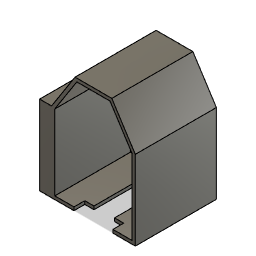
dc-15s_custom_holster (Autodesk Fusion 360 design; units mm, degrees)
Autodesk Fusion 360 part; units mm, degrees
sketch "Sketch1" plane through (0, 0, 0) normal (0, 1, 0) x (1, 0, 0)
other "Base Mesh Feature1"
other "Base Mesh Feature2"
sketch "Sketch2" plane through (0, 0, 0) normal (0, 0, 1) x (1, 0, 0)
  line L0 (-38.75, -35) -> (38.75, -35)
  line L1 (38.75, -35) -> (38.75, 35)
  line L2 (38.75, 35) -> (-38.75, 35)
  line L3 (-38.75, 35) -> (-38.75, -35)
  line L4 (-38.75, -35) -> (38.75, 35) construction
  line L5 (38.75, -35) -> (-38.75, 35) construction
  line L6 (38.75, 35) -> (-38.75, 35)
  line L7 (-38.75, 35) -> (-38.75, 47.5)
  line L8 (-38.75, 47.5) -> (38.75, 47.5)
  line L9 (38.75, 47.5) -> (38.75, 35)
  line L10 (25, 58.75) -> (-25, 58.75)
  line L11 (-25, 58.75) -> (-25, 11.25)
  line L12 (-25, 11.25) -> (25, 11.25)
  line L13 (25, 11.25) -> (25, 58.75)
  line L14 (25, 58.75) -> (-25, 11.25) construction
  line L15 (-25, 58.75) -> (25, 11.25) construction
  line L16 (17, 0.41) -> (-17, 0.41)
  line L17 (-17, 0.41) -> (-17, 69.59)
  line L18 (-17, 69.59) -> (17, 69.59)
  line L19 (17, 69.59) -> (17, 0.41)
  line L20 (17, 0.41) -> (-17, 69.59) construction
  line L21 (-17, 0.41) -> (17, 69.59) construction
  line L22 (25, 35) -> (17, 47.5)
  line L23 (-17, 47.5) -> (-25, 35)
  line L24 (38.75, -35) -> (-38.75, -35)
  line L25 (-38.75, -35) -> (-38.75, -60)
  line L26 (-38.75, -60) -> (38.75, -60)
  line L27 (38.75, -60) -> (38.75, -35)
  line L28 (-17, 47.5) -> (-38.75, 13.5156)
  line L29 (17, 47.5) -> (38.75, 13.5156)
  point P0 (0, 35)
  point P1 (0, 35)
  dimension "d1" = 77.5
  dimension "d2" = 70
  dimension "d3" = 12.5
  dimension "d4" = 50
  dimension "d5" = 47.5
  dimension "d6" = 34
  dimension "d7" = 25
  constraint horizontal L0
  constraint perpendicular L0 L1
  constraint parallel L0 L2
  constraint parallel L1 L3
  constraint coincident L4 origin
  constraint coincident L5 origin
  constraint perpendicular L6 L7
  constraint parallel L6 L8
  constraint parallel L7 L9
  constraint horizontal L10
  constraint perpendicular L10 L11
  constraint parallel L10 L12
  constraint parallel L11 L13
  constraint coincident L14 P1
  constraint coincident L15 P1
  constraint midpoint L6 P1
  constraint horizontal L16
  constraint perpendicular L16 L17
  constraint parallel L16 L18
  constraint parallel L17 L19
  constraint coincident L20 P1
  constraint coincident L21 P1
  constraint coincident P1 P0
  constraint midpoint L13 L22.start
  constraint coincident L8 L22.end
  constraint coincident L19 L22.end
  constraint coincident L8 L23.start
  constraint coincident L17 L23.start
  constraint midpoint L11 L23.end
  constraint perpendicular L24 L25
  constraint parallel L24 L26
  constraint parallel L25 L27
  constraint parallel L23 L28
  constraint coincident L1 L29.end
  constraint parallel L22 L29
  measures "d1" distance of L1.end L2.end
  measures "d2" distance of L0.end L1.end
  measures "d3" distance of L1.end L8.end
  measures "d4" distance of L11.end L12.end
  measures "d5" distance of L10.end L11.end
  measures "d6" distance of L17.end L18.end
  measures "d7" distance of L0.end L26.end
extrude "Extrude1" add sketch "Sketch2" along normal blind 5 contours L0 L1 L3 L11 L12 L13 L16 L17 L19 L24 L28 L29 | L0 L24 L25 L26 L27 | L2 L6 L17 L23 L28 | L2 L6 L11 L12 L17 | L2 L6 L12 L13 L19 | L2 L6 L19 L22 L29 | L2 L6 L8 L17 L19 | L2 L6 L12 L17 L19 | L12 L16 L17 L19
sketch "Sketch3" plane through (0, 0, 5) normal (0, 0, 1) x (1, 0, 0)
  line L0 (38.75, 13.5156) -> (17, 47.5)
  line L1 (17, 47.5) -> (-17, 47.5)
  line L2 (-17, 47.5) -> (-38.75, 13.5156)
  line L3 (-38.75, 13.5156) -> (-38.75, -60)
  line L4 (38.75, -60) -> (38.75, 13.5156)
  line L5 (-38.75, -60) -> (38.75, -60)
  line L6 (23.3582, 32) -> (15.3582, 44.5)
  line L7 (15.3582, 44.5) -> (-15.3582, 44.5)
  line L8 (-15.3582, 44.5) -> (-23.3582, 32)
  line L9 (-23.3582, 32) -> (-35.75, 32)
  line L10 (-35.75, 32) -> (-35.75, -57)
  line L11 (-35.75, -57) -> (35.75, -57)
  line L12 (35.75, -57) -> (35.75, 32)
  line L13 (35.75, 32) -> (23.3582, 32)
  line L14 (-15.3582, 44.5) -> (-35.75, 12.6378)
  line L15 (15.3582, 44.5) -> (35.75, 12.6378)
  constraint parallel L0 L6
  constraint parallel L1 L7
  constraint parallel L2 L8
  constraint parallel L3 L10
  constraint parallel L5 L11
  constraint parallel L4 L12
  constraint coincident L10 L14.end
  constraint parallel L2 L14
  constraint coincident L12 L15.end
  constraint parallel L6 L15
extrude "Extrude2" add sketch "Sketch3" along normal blind 10 contours L0 L2 L3 L4 L5 L10 L11 L12 | L0 L12 L13 L15 | L0 L1 L2 L6 L7 L8 L9 L13 L14 L15 | L2 L9 L10 L14
sketch "Sketch4" plane through (0, 0, 15) normal (0, 0, 1) x (1, 0, 0)
  line L0 (35.75, 12.6378) -> (35.75, -57)
  line L1 (35.75, -57) -> (-35.75, -57)
  line L2 (-35.75, -57) -> (-35.75, 12.6378)
  line L3 (-38.75, -60) -> (38.75, -60)
  line L4 (38.75, -60) -> (38.75, 13.5156)
  line L5 (38.75, 13.5156) -> (17, 47.5)
  line L6 (-17, 47.5) -> (-38.75, 13.5156)
  line L7 (-38.75, 13.5156) -> (-38.75, -60)
  line L8 (9.5, -63.0415) -> (-9.5, -63.0415)
  line L9 (-9.5, -63.0415) -> (-9.5, -56.9585)
  line L10 (-9.5, -56.9585) -> (9.5, -56.9585)
  line L11 (9.5, -56.9585) -> (9.5, -63.0415)
  line L12 (9.5, -63.0415) -> (-9.5, -56.9585) construction
  line L13 (-9.5, -63.0415) -> (9.5, -56.9585) construction
  line L14 (-35.75, 12.6378) -> (-15.3582, 44.5)
  line L15 (-15.3582, 44.5) -> (15.3582, 44.5)
  line L16 (15.3582, 44.5) -> (35.75, 12.6378)
  line L17 (17, 47.5) -> (-17, 47.5)
  point P0 (0, -60)
  dimension "d14" = 19
  constraint horizontal L8
  constraint perpendicular L8 L9
  constraint parallel L8 L10
  constraint parallel L9 L11
  constraint coincident L12 P0
  constraint coincident L13 P0
  constraint midpoint L3 P0
  measures "d14" distance of L9.end L10.end
extrude "Extrude3" add sketch "Sketch4" along normal blind 50 contours L0 L1 L2 L3 L4 L5 L6 L7 L9 L11 L14 L15 L16 L17
sketch "Sketch5" plane through (0, 0, 5) normal (0, 0, 1) x (1, 0, 0)
  line L0 (-35.75, 12.6378) -> (-35.75, -57)
  line L1 (-35.75, -57) -> (35.75, -57)
  line L2 (35.75, -57) -> (35.75, 12.6378)
  line L3 (-37.75, -59) -> (37.75, -59)
  line L4 (37.75, -59) -> (37.75, 34)
  line L5 (37.75, 34) -> (24.4527, 34)
  line L6 (24.4527, 34) -> (16.4527, 46.5)
  line L7 (16.4527, 46.5) -> (-16.4527, 46.5)
  line L8 (-16.4527, 46.5) -> (-24.4527, 34)
  line L9 (-24.4527, 34) -> (-37.75, 34)
  line L10 (-37.75, 34) -> (-37.75, -59)
  line L11 (14.2637, 42.5) -> (-14.2637, 42.5)
  line L12 (-14.2637, 42.5) -> (-22.2637, 30)
  line L13 (-22.2637, 30) -> (-33.75, 30)
  line L14 (-33.75, 30) -> (-33.75, -55)
  line L15 (-33.75, -55) -> (33.75, -55)
  line L16 (33.75, -55) -> (33.75, 30)
  line L17 (33.75, 30) -> (22.2637, 30)
  line L18 (22.2637, 30) -> (14.2637, 42.5)
  line L19 (35.75, 12.6378) -> (15.3582, 44.5)
  line L20 (15.3582, 44.5) -> (-15.3582, 44.5)
  line L21 (-15.3582, 44.5) -> (-35.75, 12.6378)
  constraint parallel L1 L3
  constraint parallel L2 L4
  constraint parallel L0 L10
  constraint parallel L0 L14
  constraint parallel L1 L15
  constraint parallel L2 L16
sketch "Sketch7" plane through (0, 0, 5) normal (0, 0, 1) x (1, 0, 0)
  line L0 (-35.75, 12.6378) -> (-35.75, -57)
  line L1 (-35.75, -57) -> (35.75, -57)
  line L2 (35.75, -57) -> (35.75, 12.6378)
  line L3 (35.75, 12.6378) -> (15.3582, 44.5)
  line L4 (15.3582, 44.5) -> (-15.3582, 44.5)
  line L5 (-15.3582, 44.5) -> (-35.75, 12.6378)
  line L6 (-34.25, -55.5) -> (34.25, -55.5)
  line L7 (34.25, -55.5) -> (34.25, 12.1989)
  line L8 (34.25, 12.1989) -> (14.5373, 43)
  line L9 (14.5373, 43) -> (-14.5373, 43)
  line L10 (-14.5373, 43) -> (-34.25, 12.1989)
  line L11 (-34.25, 12.1989) -> (-34.25, -55.5)
  dimension "d25" = -1.5
extrude "Extrude4" [suppressed]
sketch "Sketch6" plane through (0, 0, 65) normal (0, 0, 1) x (1, 0, 0)
  line L0 (-17, 47.5) -> (-38.75, 13.5156)
  line L1 (-38.75, 13.5156) -> (-38.75, -60)
  line L2 (9.5, -60) -> (38.75, -60)
  line L3 (-9.5, -60) -> (-9.5, -57)
  line L4 (-35.75, -57) -> (-35.75, 12.6378)
  line L5 (-9.5, -60) -> (-18, -60)
  line L6 (-18, -60) -> (-18, -57)
  line L7 (-18, -57) -> (-9.5, -57)
  line L8 (-9.5, -57) -> (-9.5, -60)
  line L9 (9.5, -58.5) -> (9.5, -60)
  line L10 (-9.5, -57) -> (-35.75, -57)
  line L11 (9.5, -57) -> (9.5, -60)
  line L12 (9.5, -60) -> (18, -60)
  line L13 (18, -60) -> (18, -57)
  line L14 (18, -57) -> (9.5, -57)
  line L15 (9.5, -57) -> (9.5, -60)
  line L16 (38.75, -60) -> (38.75, 13.5156)
  line L17 (38.75, 13.5156) -> (17, 47.5)
  line L18 (17, 47.5) -> (-17, 47.5)
  line L19 (-35.75, 12.6378) -> (-15.3582, 44.5)
  line L20 (-15.3582, 44.5) -> (15.3582, 44.5)
  line L21 (15.3582, 44.5) -> (35.75, 12.6378)
  line L22 (35.75, 12.6378) -> (35.75, -57)
  line L23 (35.75, -57) -> (9.5, -57)
  line L24 (-38.75, -60) -> (-9.5, -60)
  dimension "d21" = 8.5
  dimension "d24" = 8.5
  constraint perpendicular L5 L6
  constraint parallel L5 L7
  constraint parallel L6 L8
  constraint perpendicular L3 L5
  constraint coincident L2.end L3.start
  constraint coincident L3.end L7.end
  constraint perpendicular L11 L12
  constraint parallel L11 L13
  constraint parallel L12 L14
  measures "d21" distance of L3.start L5.end
  measures "d24" distance of L11.start L13.end
extrude "Extrude5" add sketch "Sketch6" along normal blind 10 contours L0 L1 L2 L4 L6 L10 L13 L16 L17 L18 L19 L20 L21 L22 L23 L24
extrude "Extrude6" cut sketch "Sketch7" against normal blind 5 contours L6 L7 L8 L9 L10 L11
extrude "Extrude7" add 1 faces at (-38.75, -35.4948, 50) along direction (-1, 0, 0) blind 11
sketch "Sketch8" plane through (0, -60, 0) normal (0, -1, 0) x (1, 0, 0)
  line L0 (-49.75, 0) -> (38.75, 0)
  line L1 (38.75, 0) -> (38.75, 75)
  line L2 (38.75, 75) -> (18, 75)
  line L3 (18, 75) -> (18, 65)
  line L4 (18, 65) -> (9.5, 65)
  line L5 (9.5, 65) -> (9.5, 15)
  line L6 (9.5, 15) -> (-9.5, 15)
  line L7 (-9.5, 15) -> (-9.5, 65)
  line L8 (-9.5, 65) -> (-18, 65)
  line L9 (-18, 65) -> (-18, 75)
  line L10 (-18, 75) -> (-49.75, 75)
  line L11 (-49.75, 75) -> (-49.75, 0)
  line L12 (-46.75, 3) -> (35.75, 3)
  line L13 (35.75, 3) -> (35.75, 72)
  line L14 (35.75, 72) -> (21, 72)
  line L15 (21, 72) -> (21, 62)
  line L16 (21, 62) -> (12.5, 62)
  line L17 (12.5, 62) -> (12.5, 12)
  line L18 (12.5, 12) -> (-12.5, 12)
  line L19 (-12.5, 12) -> (-12.5, 62)
  line L20 (-12.5, 62) -> (-21, 62)
  line L21 (-21, 62) -> (-21, 72)
  line L22 (-21, 72) -> (-46.75, 72)
  line L23 (-46.75, 72) -> (-46.75, 3)
  line L24 (-46.75, 3) -> (-38.75, 3)
  line L25 (-38.75, 3) -> (-38.75, 0)
  line L26 (-38.75, 0) -> (-46.75, 0)
  line L27 (-46.75, 0) -> (-46.75, 3)
  line L28 (-38.75, 3) -> (-46.75, 3)
  line L29 (-46.75, 3) -> (-46.75, 72)
  line L30 (-46.75, 72) -> (-38.75, 72)
  line L31 (-38.75, 72) -> (-38.75, 3)
  line L32 (-46.75, 37.5) -> (-38.75, 37.5)
  line L33 (-38.75, 37.5) -> (-38.75, 72)
  line L34 (-38.75, 72) -> (-46.75, 72)
  line L35 (-46.75, 72) -> (-46.75, 37.5)
  line L36 (-46.75, 3) -> (-42.75, 3)
  line L37 (-42.75, 3) -> (-42.75, 72)
  line L38 (-42.75, 72) -> (-46.75, 72)
  line L39 (-46.75, 72) -> (-46.75, 3)
  line L40 (-39.5, 20) -> (-46, 20)
  line L41 (-46, 20) -> (-46, 55)
  line L42 (-46, 55) -> (-39.5, 55)
  line L43 (-39.5, 55) -> (-39.5, 20)
  line L44 (-39.5, 20) -> (-46, 55) construction
  line L45 (-46, 20) -> (-39.5, 55) construction
  point P0 (-42.75, 37.5)
  dimension "d30" = -3
  dimension "d31" = 8
  dimension "d32" = 6.5
  dimension "d33" = 35
  constraint perpendicular L24 L25
  constraint parallel L24 L26
  constraint parallel L25 L27
  constraint perpendicular L23 L24
  constraint perpendicular L28 L29
  constraint parallel L28 L30
  constraint parallel L29 L31
  constraint perpendicular L32 L33
  constraint parallel L32 L34
  constraint parallel L33 L35
  constraint midpoint L31 L32.end
  constraint perpendicular L31 L32
  constraint midpoint L29 L32.start
  constraint perpendicular L36 L37
  constraint parallel L36 L38
  constraint parallel L37 L39
  constraint midpoint L24 L36.end
  constraint horizontal L40
  constraint perpendicular L40 L41
  constraint parallel L40 L42
  constraint parallel L41 L43
  constraint coincident L44 P0
  constraint coincident L45 P0
  constraint midpoint L32 P0
  measures "d31" distance of L12.start L24.end
  measures "d32" distance of L41.end L42.end
  measures "d33" distance of L40.end L41.end
extrude "Extrude8" cut sketch "Sketch8" against normal blind 100 contours L32 L37 L40 L41 | L32 L37 L40 L43 | L32 L37 L41 L42 | L32 L37 L42 L43
